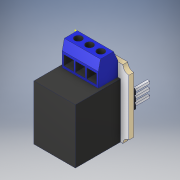
# Autodesk Inventor part: Relay
Saved by Autodesk Inventor 2019 (Build 230136000, 136)
## iProperties
Created: 2020-05-19
Part Number: Relay
Material: Пластик АБС
Document SubType Name: Modeling
Designer: Surflay
Density: 1.06 g/cm^3
Appearance: PTFE
Author: Surflay
Autodesk Inventor part; units mm, degrees
ref_plane "YZ Plane" through (0, 0, 0) normal (1, 0, 0) x (0, 1, 0)
sketch "Эскиз1" plane through (0, 0, 0) normal (0, 0, 1) x (1, 0, 0)
  line L0 (0, 0) -> (2.5, 0) construction
  line L1 (24, 0) -> (24, 2.5) construction
  line L2 (24, 28) -> (21.5, 28) construction
  line L3 (0, 28) -> (0, 25.5) construction
  arc A0 (0, 25.5) -> (2.5, 28) centre (0, 28) ccw
  arc A1 (2.5, 28) -> (0, 25.5) centre (0, 28) ccw construction
  line L4 (2.5, 28) -> (0, 28) construction
  line L5 (0, 25.5) -> (0, 2.5)
  arc A2 (21.5, 28) -> (24, 25.5) centre (24, 28) ccw
  arc A3 (24, 2.5) -> (21.5, 0) centre (24, 0) ccw
  arc A4 (2.5, 0) -> (0, 2.5) centre (0, 0) ccw
  arc A5 (0, 2.5) -> (2.5, 0) centre (0, 0) ccw construction
  arc A6 (21.5, 0) -> (24, 2.5) centre (24, 0) ccw construction
  arc A7 (24, 25.5) -> (21.5, 28) centre (24, 28) ccw construction
  line L6 (21.5, 28) -> (2.5, 28)
  line L7 (24, 25.5) -> (24, 28) construction
  line L8 (24, 2.5) -> (24, 25.5)
  line L9 (21.5, 0) -> (24, 0) construction
  line L10 (2.5, 0) -> (21.5, 0)
  line L11 (0, 2.5) -> (0, 0) construction
  dimension "d0" = 24
  dimension "d1" = 28
  dimension "d2" = 5
  dimension "d3" = 5
  dimension "d4" = 5
  dimension "d5" = 5
  constraints: 24 end point, 18 parallel, 16 point on circle, 9 perpendicular, 8 centre point, 4 coincident, 3 horizontal
  measures "d0" distance of L3.start L2.start
  measures "d1" distance of L2.start L1.start
  measures "d2" diameter of A0
  measures "d3" diameter of A2
  measures "d4" diameter of A3
  measures "d5" diameter of A4
extrude "Выдавливание1" add sketch "Эскиз1" along normal blind 2
ref_plane "РабПлоскость1" through (0, 0, 2) normal (0, 0, 1) x (1, 0, 0)
sketch "Эскиз2" plane through (0, 0, 2) normal (0, 0, 1) x (1, 0, 0)
  line L0 (3.5, 22.5) -> (20.5, 22.5)
  line L1 (20.5, 22.5) -> (20.5, 0)
  line L2 (20.5, 0) -> (3.5, 0)
  line L3 (3.5, 0) -> (3.5, 22.5)
  line L4 (2.5, 0) -> (21.5, 0) projected
  point P0 (0, 0)
  point P1 (12, 0)
  dimension "d9" = 17
  dimension "d10" = 22.5
  constraints: 8 end point, 2 midpoint, 2 parallel, 1 horizontal, 1 perpendicular
  measures "d9" distance between parallel lines of L1 L3
  measures "d10" distance between parallel lines of L2 L0
extrude "Выдавливание2" add sketch "Эскиз2" along normal blind 18.5
split body "Разделение1" result two bodies by plane through (0, 0, 2) normal (0, 0, 1) first body at (20, 15, 14.3333)
sketch "Эскиз3" plane through (3.5, 22.5, 20.5) normal (0, 1, 0) x (1, 0, 0)
  line L0 (0, 18.5) -> (17, 18.5) projected
  line L1 (15.9, 18.5) -> (1.1, 18.5)
  line L2 (1.1, 18.5) -> (1.1, 10.5)
  line L3 (1.1, 10.5) -> (15.9, 10.5)
  line L4 (15.9, 10.5) -> (15.9, 18.5)
  line L5 (0, 18.5) -> (0, 0) projected
  point P0 (-3.5, 20.5)
  dimension "d13" = 14.8
  dimension "d14" = 8
  dimension "d15" = 1.1
  constraints: 8 end point, 2 parallel, 1 horizontal, 1 perpendicular, 1 point on line
  measures "d13" distance of L3.end L2.end
  measures "d14" distance of L2.end L1.end
  measures "d15" distance between parallel lines of L5 L2
extrude "Выдавливание3" add sketch "Эскиз3" along normal blind 6 bodies 2
sketch "Эскиз4" plane through (4.6, 22.5, 10) normal (0, 0, 1) x (1, 0, 0)
  line L0 (4.7, 1) -> (0.7, 1)
  line L1 (0.7, 1) -> (0.7, 5)
  line L2 (0.7, 5) -> (4.7, 5)
  line L3 (4.7, 5) -> (4.7, 1)
  line L4 (0, 0) -> (0, 6) projected
  line L5 (0, 6) -> (14.8, 6) projected
  line L6 (14.1, 1) -> (10.1, 1)
  line L7 (10.1, 1) -> (10.1, 5)
  line L8 (10.1, 5) -> (14.1, 5)
  line L9 (14.1, 5) -> (14.1, 1)
  line L10 (14.8, 0) -> (14.8, 6) projected
  line L11 (9.4, 1) -> (5.4, 1)
  line L12 (5.4, 1) -> (5.4, 5)
  line L13 (5.4, 5) -> (9.4, 5)
  line L14 (9.4, 5) -> (9.4, 1)
  line L15 (14.8, 0) -> (0, 0) projected
  point P0 (-4.6, -22.5)
  dimension "d18" = 4
  dimension "d19" = 4
  dimension "d20" = 0.7
  dimension "d21" = 1
  dimension "d22" = 4
  dimension "d23" = 4
  dimension "d24" = 0.7
  dimension "d25" = 1
  dimension "d26" = 0.7
  dimension "d27" = 0.7
  dimension "d28" = 4
  dimension "d29" = 4
  dimension "d30" = 1
  constraints: 24 end point, 6 parallel, 3 horizontal, 3 perpendicular
  measures "d18" distance between parallel lines of L3 L1
  measures "d19" distance between parallel lines of L2 L0
  measures "d20" distance between parallel lines of L4 L1
  measures "d21" distance between parallel lines of L5 L2
  measures "d22" distance between parallel lines of L8 L6
  measures "d23" distance between parallel lines of L7 L9
  measures "d24" distance between parallel lines of L10 L9
  measures "d25" distance between parallel lines of L5 L8
  measures "d26" distance between parallel lines of L7 L14
  measures "d27" distance between parallel lines of L3 L12
  measures "d28" distance between parallel lines of L13 L11
  measures "d29" distance between parallel lines of L12 L14
  measures "d30" distance between parallel lines of L11 L15
extrude "Выдавливание4" cut sketch "Эскиз4" against normal blind 4 contours L0 L1 L2 L3 | L6 L7 L8 L9 | L11 L12 L13 L14 bodies 2
ref_plane "РабПлоскость2" through (3.5, 32.5, 20.5) normal (0, 1, 0) x (1, 0, 0)
sketch "Эскиз5" plane through (3.5, 28.5, 20.5) normal (0, 1, 0) x (1, 0, 0)
  point P0 (-3.5, 20.5)
sketch "Эскиз6" plane through (3.5, 32.5, 20.5) normal (0, 1, 0) x (1, 0, 0)
  line L0 (15.9, 18.5) -> (15.9, 10.5) projected
  line L1 (1.1, 18.5) -> (1.1, 10.5) projected
  line L2 (15.9, 11.388) -> (1.1, 11.388)
  line L3 (1.1, 11.388) -> (1.1, 16.748)
  line L4 (1.1, 16.748) -> (15.9, 16.748)
  line L5 (15.9, 16.748) -> (15.9, 11.388)
  line L6 (1.1, 10.5) -> (15.9, 10.5) projected
  point P0 (-3.5, 20.5)
  dimension "d34" = 0.888
  dimension "d35" = 5.36
  constraints: 8 end point, 2 parallel, 2 point on line, 1 horizontal, 1 perpendicular
  measures "d34" distance between parallel lines of L2 L6
  measures "d35" distance between parallel lines of L4 L2
loft "Лофт1" add profiles "Эскиз6" bodies 2 section 1 edges at (12, 28.5, 2) (4.6, 28.5, 6) (12, 28.5, 10) (19.4, 28.5, 6) contours L0 L2 L1 L4
sketch "Эскиз7" plane through (4.6, 32.5, 3.752) normal (0, 1, 0) x (1, 0, 0)
  line L0 (14.8, 0) -> (14.8, -5.36) projected
  line L1 (14.8, -5.36) -> (0, -5.36) projected
  point P0 (-4.6, 3.752)
  point P1 (12.1, -2.547)
  dimension "d40" = 2.7
  dimension "d41" = 2.813
  measures "d40" distance from line of L0 point (12.1, -2.547)
  measures "d41" distance from line of L1 point (12.1, -2.547)
hole "Отверстие1" at (16.7, 32.5, 6.299) direction (0, -1, 0) diameter 3 depth 2 bodies 2
pattern_linear "Прямоуг.массив1" count 3 spacing 4.6 along (-1, 0, 0) of "Отверстие1" bodies 2
sketch "Эскиз8" plane through (0, 0, 0) normal (0, 0, -1) x (-1, 0, 0)
  line L0 (-3.7948, 17.5) -> (-3.7948, 15.96)
  line L1 (-2.5248, 15.46) -> (-3.2948, 15.46)
  line L2 (-3.7948, 16.73) -> (-3.7948, 15.96)
  line L3 (-3.7948, 15.96) -> (-3.2948, 15.46)
  line L4 (-2.5248, 15.46) -> (-1.7548, 15.46)
  line L5 (-1.7548, 15.46) -> (-1.2548, 15.96)
  line L6 (-1.2548, 15.96) -> (-1.2548, 17.5)
  line L7 (-1.2548, 17.5) -> (-1.7548, 18)
  line L8 (-3.2948, 18) -> (-3.7948, 17.5)
  line L9 (-3.2948, 18) -> (-1.7548, 18)
  line L10 (-21.5, 28) -> (-2.5, 28) projected
  point P0 (0, 0)
  dimension "d52" = 0.77
  dimension "d53" = 0.77
  dimension "d54" = 0.77
  dimension "d55" = 1.54
  dimension "d56" = 2.54
  dimension "d57" = 2.54
  dimension "d58" = 2.885
  dimension "d59" = 2.885
  dimension "d60" = 2.54
  dimension "d61" = 2.54
  dimension "d62" = 2.54
  dimension "d63" = 10
  constraints: 20 end point, 1 horizontal, 1 midpoint, 1 perpendicular
  measures "d52" distance of L3.end L1.start
  measures "d53" distance of L2.end L2.start
  measures "d54" distance of L4.end L1.start
  measures "d55" distance of L5.end L6.end
  measures "d56" distance between parallel lines of L9 L4
  measures "d57" distance between parallel lines of L6 L0
  measures "d58" distance between parallel lines of L5 L8
  measures "d59" distance between parallel lines of L7 L3
  measures "d60" distance of L9.end L4.end
  measures "d61" distance of L0.start L6.end
  measures "d62" distance of L3.end L8.start
  measures "d63" distance between parallel lines of L10 L9
extrude "Выдавливание5" add sketch "Эскиз8" along normal blind 2 bodies 3
sketch "Эскиз9" plane through (0, 0, -2) normal (0, 0, -1) x (-1, 0, 0)
  line L0 (-2.0248, 17.23) -> (-3.0248, 17.23)
  line L1 (-3.0248, 17.23) -> (-3.0248, 16.23)
  line L2 (-3.0248, 16.23) -> (-2.0248, 16.23)
  line L3 (-2.0248, 16.23) -> (-2.0248, 17.23)
  line L4 (-1.2548, 15.96) -> (-1.2548, 17.5) projected
  line L5 (-3.2948, 15.46) -> (-1.7548, 15.46) projected
  point P0 (0, 0)
  dimension "d66" = 1
  dimension "d67" = 1
  dimension "d68" = 0.77
  dimension "d69" = 0.77
  constraints: 8 end point, 2 parallel, 1 horizontal, 1 perpendicular
  measures "d66" distance between parallel lines of L2 L0
  measures "d67" distance between parallel lines of L1 L3
  measures "d68" distance between parallel lines of L4 L3
  measures "d69" distance between parallel lines of L2 L5
extrude "Выдавливание6" add sketch "Эскиз9" along normal blind 6.5 bodies 3
pattern_linear "Прямоуг.массив2" count 3 spacing 2.54 along (0, -1, 0) of "Выдавливание5", "Выдавливание6" bodies 3
pattern_linear "Прямоуг.массив3" count 2 spacing -19 along (-1, 0, 0) of "Выдавливание5", "Выдавливание6", "Прямоуг.массив2" bodies 3
